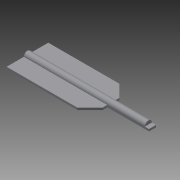
# Autodesk Inventor part: current-adjusting-screwdriver
Saved by Autodesk Inventor 2014 (Build 180170000, 170)
## iProperties
Created: 2014-11-01
Part Number: current-adjusting-screwdriver
Material: Generic
Document SubType Name: Modeling
Designer: caleb
Density: 1 g/cm^3
Appearance: Default
Author: caleb
Autodesk Inventor part; units mm, degrees
ref_plane "YZ Plane" through (0, 0, 0) normal (1, 0, 0) x (0, 1, 0)
ref_plane "XZ Plane" through (0, 0, 0) normal (0, 1, 0) x (-1, 0, 0)
sketch "Sketch5" plane through (0, 0, 0) normal (0, 0, 1) x (1, 0, 0)
  line L0 (0, 0) -> (20, 0)
  line L1 (20, 0) -> (20, 10)
  line L2 (20, 10) -> (0, 10)
  line L3 (0, 10) -> (0, 0)
  line L4 (20, 4.15) -> (30, 4.15)
  line L5 (30, 4.15) -> (30, 5.85)
  line L6 (30, 5.85) -> (20, 5.85)
  line L7 (20, 5.85) -> (20, 4.15)
  point P0 (20, 5)
  point P1 (20, 5)
  dimension "d11" = 10
  dimension "d12" = 1.7
  dimension "d13" = 20
  dimension "d14" = 10
  constraints: 16 end point, 4 parallel, 2 horizontal, 2 midpoint, 2 perpendicular, 1 coincident, 1 point on line
  measures "d11" distance of L2.end L0.start
  measures "d12" distance of L4.end L5.end
  measures "d13" distance of L0.start L0.end
  measures "d14" distance of L4.start L4.end
extrude "Extrusion3" add sketch "Sketch5" along normal blind 0.5
chamfer "Chamfer1" distance 3 angle 45 2 edges at (20, 10, 0.25) (20, 0, 0.25)
ref_plane "Work Plane1" through (29, 4.15, 0) normal (1, 0, 0) x (0, 0, -1)
sketch "Sketch6" plane through (29, 4.15, 0) normal (1, 0, 0) x (0, 0, -1)
  line L0 (0, 1.7) -> (0, 0) projected
  line L1 (0, 0) -> (-0.5, 0) projected
  line L2 (-0.5, 0) -> (-0.5, 1.7) projected
  line L3 (-0.5, 1.7) -> (0, 1.7) projected
  arc A0 (-0.5, 1.7) -> (-0.5, 0) centre (-0.5, 0.85) ccw
  point P0 (0, -4.15)
  constraints: 2 point on circle, 2 tangent, 1 centre point
extrude "Extrusion4" add sketch "Sketch6" against normal up to surface (29 mm away) contours L2 A0
body "Solid2"
